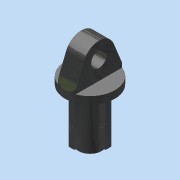
# Autodesk Inventor part: Shock Mount - Bottom
Saved by Autodesk Inventor 2011 SP1 (Build 150282100, 282)
## iProperties
Created: 2011-09-22
Part Number: Shock Mount - Bottom
Document SubType Name: Modeling
Designer: dgitz
Density: 1 g/cm^3
Author: dgitz
Autodesk Inventor part; units mm, degrees
ref_plane "YZ Plane" through (0, 0, 0) normal (1, 0, 0) x (0, 1, 0)
ref_plane "XZ Plane" through (0, 0, 0) normal (0, 1, 0) x (-1, 0, 0)
ref_plane "XY Plane" through (0, 0, 0) normal (0, 0, 1) x (1, 0, 0)
sketch "Sketch8" plane through (0, 0, 0) normal (0, 1, 0) x (-1, 0, 0)
  circle A0 centre (0, 0) radius 8.509
  dimension "d28" = 17.018
  constraints: 1 centre point, 1 coincident
  measures "d28" diameter of A0
extrude "Extrusion7" add sketch "Sketch8" along normal blind 2.54
sketch "Sketch9" plane through (0, 0, 0) normal (1, 0, 0) x (0, 1, 0)
  line L0 (0, 8.509) -> (2.54, 8.509) projected
  line L1 (2.54, 8.509) -> (2.54, -8.509) projected
  line L2 (0, -8.509) -> (2.54, -8.509) projected
  line L3 (2.54, 8.509) -> (2.54, -8.509)
  line L4 (2.54, -8.509) -> (11.0639, -5.0629)
  line L5 (2.54, 8.509) -> (11.0639, 5.0629)
  arc A0 (11.0639, -5.0629) -> (11.0639, 5.0629) centre (9.017, 0) ccw
  circle A1 centre (9.017, 0) radius 2.667
  line L6 (-3.0224, 0) -> (5.6412, 0) construction
  line L7 (14.478, 5.5398) -> (14.478, 0.9968) construction
  point P0 (0, 0)
  dimension "d31" = 10.922
  dimension "d32" = 5.334
  dimension "d33" = 11.938
  constraints: 10 end point, 3 tangent, 2 centre point, 2 point on circle, 2 point on line, 1 coincident, 1 collinear, 1 perpendicular, 1 vertical
  measures "d31" diameter of A0
  measures "d32" diameter of A1
  measures "d33" distance between parallel lines of L1 L7
extrude "Extrusion8" add sketch "Sketch9" along normal mid plane 6.096
sketch "Sketch10" plane through (0, 2.54, 0) normal (0, 1, 0) x (1, 0, 0)
  arc A0 (3.048, -7.9444) -> (3.048, 7.9444) centre (0, 0) ccw projected
  circle A1 centre (0, 0) radius 8.509
  circle A2 centre (0, 0) radius 9.0384
  arc A3 (-3.048, 7.9444) -> (-3.048, -7.9444) centre (0, 0) ccw projected
  point P0 (-3.048, 8.509)
  constraints: 2 coincident, 1 centre point, 1 concentric, 3 other
extrude "Extrusion9" cut sketch "Sketch10" along normal blind 12.7
sketch "Sketch11" plane through (0, 0, 0) normal (0, -1, 0) x (1, 0, 0)
  circle A0 centre (0, 0) radius 8.509 projected
  circle A1 centre (0, 0) radius 1.9812
  arc A2 (-6.2682, 1.016) -> (-6.2682, -1.016) centre (0, 0) ccw
  line L0 (-6.2682, 1.016) -> (-4.3273, 1.016)
  line L1 (-6.2682, -1.016) -> (-4.3273, -1.016)
  arc A3 (-1.016, -6.2682) -> (1.016, -6.2682) centre (0, 0) ccw
  line L2 (-1.016, -6.2682) -> (-1.016, -4.3273)
  line L3 (1.016, -6.2682) -> (1.016, -4.3273)
  arc A4 (6.2682, -1.016) -> (6.2682, 1.016) centre (0, 0) ccw
  line L4 (6.2682, -1.016) -> (4.3273, -1.016)
  line L5 (6.2682, 1.016) -> (4.3273, 1.016)
  arc A5 (1.016, 6.2682) -> (-1.016, 6.2682) centre (0, 0) ccw
  line L6 (1.016, 6.2682) -> (1.016, 4.3273)
  line L7 (-1.016, 6.2682) -> (-1.016, 4.3273)
  arc A6 (-1.016, 4.3273) -> (-4.3273, 1.016) centre (0, 0) ccw
  arc A7 (4.3273, 1.016) -> (1.016, 4.3273) centre (0, 0) ccw
  arc A8 (-4.3273, -1.016) -> (-1.016, -4.3273) centre (0, 0) ccw
  arc A9 (1.016, -4.3273) -> (4.3273, -1.016) centre (0, 0) ccw
  dimension "d38" = 3.9624
  dimension "d40" = 12.7
  dimension "d41" = 2.032
  dimension "d42" = 1.016
  dimension "d45" = 360
  constraints: 16 end point, 16 point on circle, 9 centre point, 3 coincident, 1 horizontal, 1 parallel, 33 other
  measures "d38" diameter of A1
  measures "d40" diameter of A2
  measures "d41" distance between parallel lines of L1 L0
  measures "d42" distance from line of A0.centre L1
extrude "Extrusion10" add sketch "Sketch11" along normal blind 15.748 contours L0 A6 L7 A5 L6 A7 L5 A4 L4 A9 L3 A3 L2 A8 L1 A2
sketch "Sketch12" plane through (0, -15.748, 0) normal (0, -1, 0) x (1, 0, 0)
  circle A0 centre (0, 0) radius 1.9812 projected
  arc A1 (1.016, 6.2682) -> (-1.016, 6.2682) centre (0, 0) ccw projected
  circle A2 centre (0, 0) radius 1.9812
  circle A3 centre (0, 0) radius 3.937
  dimension "d49" = 7.874
  constraints: 2 centre point, 2 coincident, 1 concentric
  measures "d49" diameter of A3
extrude "Extrusion11" add sketch "Sketch12" along normal blind 2.032
body "Solid2"
